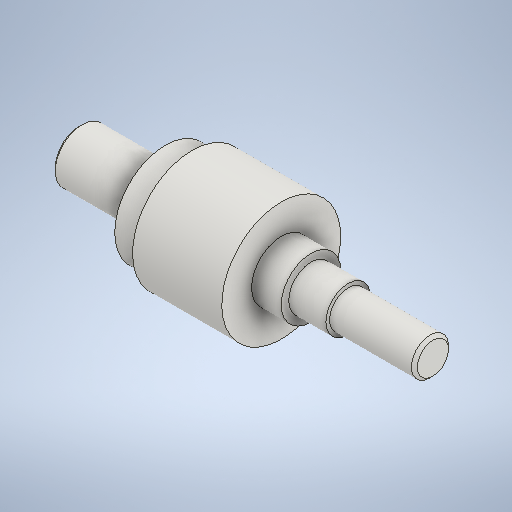
# Autodesk Inventor part: Shaft
Saved by Autodesk Inventor 2025.2 (Build 292293000, 293)
## iProperties
CustomPartVersion: 1
Created: 2024-11-26
Part Number: Shaft
Material: Steel
Document SubType Name: Modeling
Designer: hongquan
Density: 1 g/cm^3
Appearance: Steel
Length: 238.000 mm
Author: hongquan
Autodesk Inventor part; units mm, degrees
ref_plane "Start Plane" through (0, 0, 0) normal (1, 0, 0) x (0, 1, 0)
ref_plane "XZ Plane" through (0, 0, 0) normal (0, 1, 0) x (-1, 0, 0)
ref_plane "XY Plane" through (0, 0, 0) normal (0, 0, 1) x (1, 0, 0)
sketch "Main Sketch" plane through (0, 0, 0) normal (0, 0, 1) x (1, 0, 0)
  line L0 (0, 0) -> (238, 0)
  line L1 (0, 0) -> (0, 18)
  line L2 (0, 18) -> (58, 18)
  line L3 (58, 18) -> (58, 34)
  line L4 (76, 34) -> (76, 40)
  line L5 (58, 34) -> (76, 34)
  line L6 (136, 40) -> (136, 20)
  line L7 (76, 40) -> (136, 40)
  line L8 (156, 20) -> (156, 15)
  line L9 (136, 20) -> (156, 20)
  line L10 (181, 15) -> (181, 12.5)
  line L11 (156, 15) -> (181, 15)
  line L12 (238, 12.5) -> (238, 0)
  line L13 (181, 12.5) -> (238, 12.5)
  dimension "d3" = 36
  dimension "d4" = 68
  dimension "d5" = 80
  dimension "d6" = 40
  dimension "d7" = 30
  dimension "d8" = 25
  constraints: 28 end point, 7 vertical, 5 horizontal
  measures "d3" diameter of L2 L0
  measures "d4" diameter of L5 L0
  measures "d5" diameter of L7 L0
  measures "d6" diameter of L9 L0
  measures "d7" diameter of L11 L0
  measures "d8" diameter of L13 L0
revolve "Revolution1" add sketch "Main Sketch" angle 360 about axis through (0, 0, 0) along (1, 0, 0)
chamfer "Chamfer1" distance 2 angle 45 1 edges at (0, -18, 0) measured on face at (0.5, -18, 0)
chamfer "Chamfer2" distance 2 angle 45 1 edges at (238, -12.5, 0) measured on face at (237.5, -12.5, 0)
equation "\"Length\" = 238"
body "Solid1"
